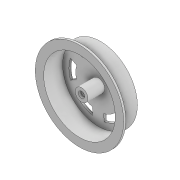
# Autodesk Inventor part: mask_breath_top
Saved by Autodesk Inventor 2021 (Build 250183000, 183)
## iProperties
Created: 2020-04-12
Part Number: mask_breath_top
Material: Generic
Document SubType Name: Modeling
Designer: Muchiri John
Density: 1 g/cm^3
Appearance: Default
Author: Muchiri John
Autodesk Inventor part; units mm, degrees
ref_plane "YZ Plane" through (0, 0, 0) normal (1, 0, 0) x (0, 1, 0)
ref_plane "XZ Plane" through (0, 0, 0) normal (0, 1, 0) x (-1, 0, 0)
ref_plane "XY Plane" through (0, 0, 0) normal (0, 0, 1) x (1, 0, 0)
sketch "Sketch1" plane through (0, 0, 0) normal (0, 0, 1) x (1, 0, 0)
  circle A0 centre (27.386, 18.5258) radius 21
  circle A1 centre (27.386, 18.5258) radius 17
  dimension "d0" = 42
  dimension "d1" = 34
  constraints: 2 centre point, 1 coincident
  measures "d0" diameter of A0
  measures "d1" diameter of A1
extrude "Outer" add sketch "Sketch1" along normal blind 1
sketch "Sketch2" plane through (27.386, 18.5258, 1) normal (0, 0, 1) x (1, 0, 0)
  circle A0 centre (0, 0) radius 17.5
  dimension "d4" = 35
  constraints: 1 centre point
  measures "d4" diameter of A0
extrude "Breath_ext_outer" add sketch "Sketch2" against normal blind 10
sketch "Sketch3" plane through (27.386, 18.5258, 1) normal (0, 0, 1) x (1, 0, 0)
  circle A0 centre (0, 0) radius 17
  dimension "d7" = 34
  constraints: 1 centre point
  measures "d7" diameter of A0
extrude "Breath_ext_inner" cut sketch "Sketch3" against normal blind 9
sketch "Sketch4" plane through (27.386, 18.5258, -9) normal (0, 0, -1) x (-1, 0, 0)
  arc A0 (-10.3804, 2.7946) -> (-10.3234, -2.9983) centre (0, 0) ccw
  arc A1 (-13.233, 4.5704) -> (-13.2519, -4.5152) centre (0, 0) ccw
  line L0 (-10.3234, -2.9983) -> (-13.2519, -4.5152)
  line L1 (-10.3804, 2.7946) -> (-13.233, 4.5704)
  arc A2 (-2.7701, 10.387) -> (-7.7583, 7.4412) centre (0, 0) ccw
  arc A3 (-2.6584, 13.7453) -> (-10.5362, 9.2189) centre (0, 0) ccw
  line L2 (-7.7583, 7.4412) -> (-10.5362, 9.2189)
  line L3 (-2.7701, 10.387) -> (-2.6584, 13.7453)
  arc A4 (7.6104, 7.5924) -> (2.5651, 10.4395) centre (0, 0) ccw
  arc A5 (10.5746, 9.1749) -> (2.7157, 13.7341) centre (0, 0) ccw
  line L4 (2.5651, 10.4395) -> (2.7157, 13.7341)
  line L5 (7.6104, 7.5924) -> (10.5746, 9.1749)
  arc A6 (10.3804, -2.7946) -> (10.3234, 2.9983) centre (0, 0) ccw
  arc A7 (13.233, -4.5704) -> (13.2519, 4.5152) centre (0, 0) ccw
  line L6 (10.3234, 2.9983) -> (13.2519, 4.5152)
  line L7 (10.3804, -2.7946) -> (13.233, -4.5704)
  arc A8 (2.7701, -10.387) -> (7.7583, -7.4412) centre (0, 0) ccw
  arc A9 (2.6584, -13.7453) -> (10.5362, -9.2189) centre (0, 0) ccw
  line L8 (7.7583, -7.4412) -> (10.5362, -9.2189)
  line L9 (2.7701, -10.387) -> (2.6584, -13.7453)
  arc A10 (-7.6104, -7.5924) -> (-2.5651, -10.4395) centre (0, 0) ccw
  arc A11 (-10.5746, -9.1749) -> (-2.7157, -13.7341) centre (0, 0) ccw
  line L10 (-2.5651, -10.4395) -> (-2.7157, -13.7341)
  line L11 (-7.6104, -7.5924) -> (-10.5746, -9.1749)
  dimension "d14" = 360
  constraints: 24 end point, 24 point on circle, 12 centre point, 8 coincident, 59 other
extrude "Breath_Holes" cut sketch "Sketch4" against normal blind 2
sketch "Sketch5" plane through (27.386, 18.5258, -8) normal (0, 0, 1) x (1, 0, 0)
  circle A0 centre (0, 0) radius 3
  dimension "d18" = 6
  constraints: 1 centre point
  measures "d18" diameter of A0
extrude "Hole_holder" add sketch "Sketch5" along normal blind 8
sketch "Sketch6" plane through (27.386, 18.5258, 0) normal (0, 0, 1) x (1, 0, 0)
  point P0 (0, 0.0702)
hole "Hole1" at (27.386, 18.596, 0) direction (0, 0, -1) diameter 2.1 depth 7 tip angle 118 counterbore diameter 3 counterbore depth 1
body "Solid1"
